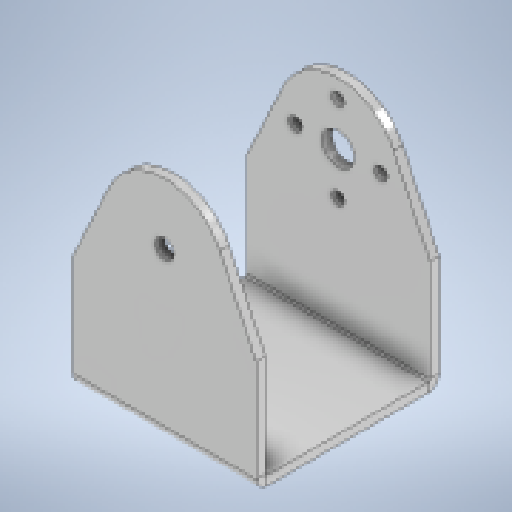
# Autodesk Inventor part: partpart
Saved by Autodesk Inventor 2025.2 (Build 292293000, 293)
## iProperties
Created: 2025-07-22
Part Number: partpart
Material: Aluminum 6061-AHC
Document SubType Name: Sheet Metal
Designer: User
Density: 2.7 g/cm^3
Sheet Metal Rule: Default_mm
Appearance: Aluminum - Dark
Author: User
Autodesk Inventor part; units mm, degrees
ref_plane "YZ Plane" through (0, 0, 0) normal (1, 0, 0) x (0, 1, 0)
ref_plane "XZ Plane" through (0, 0, 0) normal (0, 1, 0) x (-1, 0, 0)
ref_plane "XY Plane" through (0, 0, 0) normal (0, 0, 1) x (1, 0, 0)
sketch "Sketch1" plane through (0, 0, 0) normal (0, 1, 0) x (-1, 0, 0)
  line L0 (15, 14.965) -> (-15, 14.965)
  line L1 (-15, 14.965) -> (-15, -14.965)
  line L2 (-15, -14.965) -> (15, -14.965)
  line L3 (15, -14.965) -> (15, 14.965)
  point P0 (0, 0)
  dimension "d0" = 29.93
  dimension "d1" = 30
  dimension "d2" = 15
  dimension "d3" = 14.965
  measures "d0" distance of L2.end L0.start
  measures "d1" distance of L0.start L0.end
  measures "d2" distance from line of point (0, 0) L3
  measures "d3" distance from line of point (0, 0) L2
extrude "Plate1" add sketch "Sketch1" along normal blind 1.5
sketch "Sketch2" plane through (-15, 0, -13.465) normal (0, 0, -1) x (-1, 0, 0)
  line L0 (-30, 0) -> (0, 0)
  line L1 (0, 0) -> (0, 37)
  line L2 (0, 37) -> (-30, 37)
  line L3 (-30, 37) -> (-30, 0)
  constraints: 6 end point, 1 horizontal, 1 perpendicular, 1 vertical
edge flange "Flange1" height 37 angle 90 thickness 1.5 bend radius 0.31 thickness toward (0, 0, -1) relief straight relief width 1.5 relief depth 0.75 corner gap 0.31 corner form 0 edges at (0, 1.5, -14.965) (0, 1.5, 14.965) wall of the first edge with corners at (15, 0, -13.465) (-15, 0, -13.465) (-15, 37, -13.465) (15, 37, -13.465)
bend "Bend1"
corner "Corner1"
sketch "Sketch3" plane through (-15, 37, 14.965) normal (0, 0, 1) x (1, 0, 0)
  line L0 (0, 0) -> (30, 0) projected
  line L1 (0, -35.19) -> (0, 0) projected
  circle A0 centre (15, -10) radius 10
  line L2 (0, -18.5) -> (30, -18.5)
  line L3 (30, -18.5) -> (30, -28.5)
  line L4 (30, -28.5) -> (0, -28.5)
  line L5 (0, -28.5) -> (0, -18.5)
  line L6 (30, -18.5) -> (24.0624, -5.7723)
  line L7 (0, -18.5) -> (5.9376, -5.7723)
  line L8 (0, 0) -> (30, 0)
  line L9 (30, 0) -> (30, -25)
  line L10 (30, -25) -> (0, -25)
  line L11 (0, -25) -> (0, 0)
  point P0 (15, -37)
  point P1 (15, 0)
  dimension "d15" = 10
  dimension "d16" = 0
  dimension "d17" = 20
  dimension "d18" = 8.5
  dimension "d19" = 0
  dimension "d20" = 30
  dimension "d21" = 10
  dimension "d22" = 25
  constraints: 20 end point, 4 parallel, 2 horizontal, 2 perpendicular, 2 point on circle, 2 tangent, 1 centre point, 1 point on line
  measures "d15" distance from line of L0 A0.centre
  measures "d16" horizontal distance of point (15, -37) A0.centre
  measures "d17" diameter of A0
  measures "d18" distance from line of A0.centre L2
  measures "d19" distance between parallel lines of L1 L5
  measures "d20" distance of L3.end L4.end
  measures "d21" distance between parallel lines of L2 L4
  measures "d22" distance between parallel lines of L0 L10
extrude "Extrusion1" cut sketch "Sketch3" against normal blind 35 contours L0 A0 L7 L1 | L0 L9 L6 A0
sketch "Sketch4" plane through (15, 1.81, -14.965) normal (0, 0, -1) x (-1, 0, 0)
  arc A0 (24.0624, 29.4177) -> (5.9376, 29.4177) centre (15, 25.19) ccw projected
  circle A1 centre (15, 25.19) radius 2.6
  circle A2 centre (8, 25.19) radius 1.05
  circle A3 centre (22, 25.19) radius 1.05
  circle A4 centre (15, 32.19) radius 1.05
  circle A5 centre (15, 18.19) radius 1.05
  point P0 (15, -1.81)
  dimension "d25" = 5.2
  dimension "d26" = 0
  dimension "d27" = 7
  dimension "d28" = 2.1
  dimension "d29" = 7
  dimension "d30" = 0
  dimension "d31" = 2.1
  dimension "d32" = 0
  dimension "d33" = 7
  dimension "d34" = 2.1
  dimension "d35" = 7
  dimension "d36" = 0
  dimension "d37" = 2.1
  constraints: 5 centre point, 1 coincident
  measures "d25" diameter of A1
  measures "d26" vertical distance of A0.centre A2.centre
  measures "d27" distance of A0.centre A2.centre
  measures "d28" diameter of A2
  measures "d29" distance of A4.centre A0.centre
  measures "d30" horizontal distance of A0.centre A4.centre
  measures "d31" diameter of A4
  measures "d32" vertical distance of A0.centre A3.centre
  measures "d33" distance of A0.centre A3.centre
  measures "d34" diameter of A3
  measures "d35" distance of A0.centre A5.centre
  measures "d36" horizontal distance of A0.centre A5.centre
  measures "d37" diameter of A5
extrude "Extrusion2" cut sketch "Sketch4" against normal blind 1.5
sketch "Sketch5" plane through (-15, 1.81, 14.965) normal (0, 0, 1) x (1, 0, 0)
  arc A0 (24.0624, 29.4177) -> (5.9376, 29.4177) centre (15, 25.19) ccw projected
  circle A1 centre (15, 25.19) radius 1.5
  point P0 (15, -1.81)
  dimension "d40" = 3
  constraints: 1 centre point, 1 coincident
  measures "d40" diameter of A1
extrude "Extrusion3" cut sketch "Sketch5" against normal blind 1.5
equation "\"d4\" = Thickness"
equation "\"d5\" = BendReliefWidth"
equation "\"d6\" = BendReliefDepth"
equation "\"d7\" = MinimumRemnant"
equation "\"d8\" = TransitionRadius"
equation "\"d11\" = BendRadius"
equation "\"d12\" = CornerReliefSize"
equation "\"d13\" = GapSize"
equation "\"d14\" = JacobiRadiusSize"
equation "\"BendReliefWidth\" = Thickness"
equation "\"BendReliefDepth\" = 0.5 * Thickness"
equation "\"CornerReliefSize\" = 4 * Thickness"
equation "\"MinimumRemnant\" = 2 * Thickness"
equation "\"TransitionRadius\" = BendRadius"
equation "\"JacobiRadiusSize\" = BendRadius"
equation "\"GapSize\" = Thickness"
equation "\"Thickness\" = 1.5"
equation "\"BendRadius\" = 0.31"
body "Solid1"
